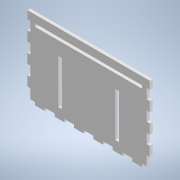
# Autodesk Inventor part: side
Saved by Autodesk Inventor 2022 (Build 260153070, 153G)
## iProperties
Created: 2022-05-11
Part Number: side
Material: Generic
Document SubType Name: Modeling
Designer: Jeanette Guo
Density: 1 g/cm^3
Appearance: Default
Author: Jeanette Guo
Autodesk Inventor part; units mm, degrees
ref_plane "YZ Plane" through (0, 0, 0) normal (1, 0, 0) x (0, 1, 0)
ref_plane "XZ Plane" through (0, 0, 0) normal (0, 1, 0) x (-1, 0, 0)
ref_plane "XY Plane" through (0, 0, 0) normal (0, 0, 1) x (1, 0, 0)
ref_plane "Work Plane2" through (0, 0, 0) normal (0, 0, 1) x (1, 0, 0)
sketch "Sketch2" plane through (0, 0, 0) normal (0, 0, 1) x (1, 0, 0)
  line L0 (-13, 0) -> (-13, 3) projected
  line L1 (-13, 3) -> (-10, 3) projected
  line L2 (103, 0) -> (103, 3) projected
  line L3 (100, 3) -> (103, 3) projected
  line L4 (103, 8) -> (-13, 8)
  line L5 (-10, 0) -> (-10, 3) projected
  line L6 (-10, 3) -> (0, 3) projected
  line L7 (100, 0) -> (100, 3) projected
  line L8 (90, 3) -> (100, 3) projected
  line L9 (0, 0) -> (0, 3) projected
  line L10 (90, 0) -> (90, 3) projected
  line L11 (90, 3) -> (90, 0)
  line L12 (0, 3) -> (0, 0)
  line L13 (45, 0) -> (45, -20) construction
  line L14 (-15.0005, 0) -> (-15.0005, -10)
  line L15 (-15.0005, -10) -> (-18.0005, -10)
  line L16 (-15.0005, -20) -> (-18.0005, -20)
  line L17 (-15.0005, -20) -> (-15.0005, -30)
  line L18 (-15.0005, -30) -> (-18.0005, -30)
  line L19 (-15.0005, -40) -> (-18.0005, -40)
  line L20 (-15.0005, -50) -> (-18.0005, -50)
  line L21 (-15.0005, -60) -> (-18.0005, -60)
  line L22 (-18.0005, -10) -> (-18.0005, -20)
  line L23 (-18.0005, -30) -> (-18.0005, -40)
  line L24 (-18.0005, -50) -> (-18.0005, -60)
  line L25 (-15.0005, -40) -> (-15.0005, -50)
  line L26 (90, -73) -> (90, -70)
  line L27 (80, -73) -> (70, -73)
  line L28 (60, -73) -> (50, -73)
  line L29 (45, -70) -> (45, -47.72) construction
  line L30 (80, -73) -> (80, -70)
  line L31 (70, -73) -> (70, -70)
  line L32 (60, -73) -> (60, -70)
  line L33 (90, -70) -> (80, -70)
  line L34 (80, -73) -> (70, -73)
  line L35 (70, -70) -> (60, -70)
  line L36 (-10, -73) -> (0, -73)
  line L37 (0, -73) -> (0, -70)
  line L38 (10, -73) -> (20, -73)
  line L39 (10, -73) -> (10, -70)
  line L40 (20, -73) -> (20, -70)
  line L41 (30, -73) -> (30, -70)
  line L42 (0, -70) -> (10, -70)
  line L43 (20, -70) -> (30, -70)
  line L44 (60, -73) -> (50, -73)
  line L45 (50, -73) -> (50, -70)
  line L46 (50, -70) -> (45, -70)
  line L47 (45, -70) -> (40, -70)
  line L48 (40, -70) -> (40, -73)
  line L49 (30, -73) -> (40, -73)
  line L50 (50, -73) -> (77.2719, -73)
  line L51 (60, -73) -> (50, -73)
  line L52 (45, -70) -> (40, -70)
  line L53 (40, -73) -> (30, -73)
  line L54 (30, -70) -> (20, -70)
  line L55 (10, -70) -> (0, -70)
  line L56 (20, -73) -> (10, -73)
  line L57 (0, -73) -> (12.7281, -73)
  line L58 (-18, 8) -> (-13, 8)
  line L59 (-15.0005, 0) -> (-18, 0)
  line L60 (-15.0005, -60) -> (-15.0005, -70)
  line L61 (-18, -50) -> (-18, -60)
  line L62 (-18, -30) -> (-18, -40)
  line L63 (-18, 8) -> (-18, 0)
  line L64 (-18, -10) -> (-18, -20)
  line L65 (105.0005, 0) -> (105.0005, -10)
  line L66 (108.0005, -10) -> (108.0005, -20)
  line L67 (105.0005, -10) -> (108.0005, -10)
  line L68 (105.0005, -20) -> (108.0005, -20)
  line L69 (105.0005, -20) -> (105.0005, -30)
  line L70 (105.0005, -30) -> (108.0005, -30)
  line L71 (108.0005, -30) -> (108.0005, -40)
  line L72 (105.0005, -40) -> (108.0005, -40)
  line L73 (105.0005, -40) -> (105.0005, -50)
  line L74 (105.0005, -50) -> (108.0005, -50)
  line L75 (108.0005, -50) -> (108.0005, -60)
  line L76 (105.0005, -60) -> (108.0005, -60)
  line L77 (108, 8) -> (103, 8)
  line L78 (105.0005, 0) -> (108, 0)
  line L79 (105.0005, -60) -> (105.0005, -70)
  line L80 (108, -50) -> (108, -60)
  line L81 (108, -30) -> (108, -40)
  line L82 (108, 8) -> (108, 0)
  line L83 (108, -10) -> (108, -20)
  line L84 (100, -73) -> (90, -73)
  line L85 (0, -73) -> (-10, -73)
  line L86 (-10, -73) -> (-10, -70)
  line L87 (-10, -70) -> (-15.0005, -70)
  line L88 (-13, -73) -> (-10, -73)
  line L89 (100, -73) -> (98, -73)
  line L90 (90, -70) -> (100, -70)
  line L91 (100, -70) -> (100, -73)
  line L92 (105.0005, -70) -> (100, -70)
  line L93 (-10, 0) -> (100, 0)
  line L94 (-10, 0) -> (-10, -3)
  line L95 (-10, -3) -> (100, -3)
  line L96 (100, -3) -> (100, 0)
  dimension "d39" = 10
  dimension "d42" = 10
  dimension "d45" = 3
  constraints: 174 end point, 32 symmetric about line, 30 perpendicular, 25 parallel, 16 point on line, 9 vertical, 7 collinear, 4 horizontal, 1 other
  measures "d39" distance of L36.end L36.start
  measures "d42" distance of L26.end L90.end
  measures "d45" distance of L5.start L94.end
extrude "Extrusion1" add sketch "Sketch2" along normal blind 3 contours L77 L82 L78 L65 L67 L66 L68 L69 L70 L71 L72 L73 L74 L75 L76 L79 L92 L90 L33 L30 L27 L31 L35 L32 L28 L45 L46 L47 L48 L49 L41 L43 L40 L38 L39 L42 L37 L36 L86 L87 L60 L21 L24 L20 L25 L19 L23 L18 L17 L16 L22 L15 L14 L59 L63 L58 L4 | L91 L84 L26 L90 | L5 L6 L9 L93 | L10 L8 L7 L93
sketch "Sketch3" plane through (0, 0, 3) normal (0, 0, 1) x (1, 0, 0)
  line L0 (105.0005, -70) -> (105.0005, -60) projected
  line L1 (-15.0005, -60) -> (-15.0005, -70) projected
  line L2 (-15.0005, -62.5302) -> (105.0005, -62.5302)
  line L3 (45, -62.5302) -> (72.5, -62.5302)
  line L4 (72.5, -67) -> (76.2143, -67)
  line L5 (76.2143, -67) -> (76.2143, -17)
  line L6 (76.2143, -17) -> (72.5, -17)
  line L7 (72.5, -17) -> (72.5, -67)
  line L8 (60, -70) -> (70, -70) projected
  line L9 (45, -62.5302) -> (45, -53.8284)
  line L10 (17.5, -67) -> (13.7857, -67)
  line L11 (13.7857, -67) -> (13.7857, -17)
  line L12 (13.7857, -17) -> (17.5, -17)
  line L13 (17.5, -17) -> (17.5, -67)
  point P0 (0, 0)
  point P1 (76.2143, -62.5302)
  point P2 (13.7857, -62.5302)
  point P3 (17.5, -62.5302)
  dimension "d47" = 27.5
  dimension "d48" = 50
  dimension "d49" = 3
  constraints: 22 end point, 4 symmetric about line, 3 point on line, 2 parallel, 2 perpendicular, 1 horizontal, 1 midpoint, 1 vertical
  measures "d47" distance of L3.start L3.end
  measures "d48" distance of L5.end L4.end
  measures "d49" distance between parallel lines of L8 L4
extrude "Extrusion2" cut sketch "Sketch3" against normal through all contours L7 L6 L5 L2 | L2 L11 L12 L13
body "Solid1"
